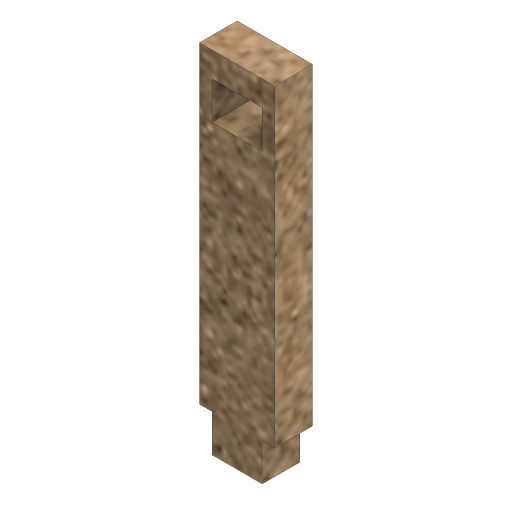
# Autodesk Inventor part: final_side
Saved by Autodesk Inventor 2024 (Build 280153000, 153)
## iProperties
Created: 2024-05-27
Material: MDF Medium Density Fiberboard
Document SubType Name: Modeling
Designer: op04o
Density: 0.8 g/cm^3
Appearance: Cardboard - Corrugated
Mass: 0.36 g
Surface Area: 5.46 cm^2
Volume: 0.45 cm^3
Author: 第26組
Title: final_side
Autodesk Inventor part; units mm, degrees
ref_plane "YZ Plane" through (0, 0, 0) normal (1, 0, 0) x (0, 1, 0)
ref_plane "XZ Plane" through (0, 0, 0) normal (0, 1, 0) x (-1, 0, 0)
ref_plane "XY Plane" through (0, 0, 0) normal (0, 0, 1) x (1, 0, 0)
sketch "Sketch1" plane through (0, 0, 0) normal (0, 0, 1) x (1, 0, 0)
  line L0 (-3, -12.5) -> (3, -12.5)
  line L1 (3, -12.5) -> (3, 12.5)
  line L2 (3, 12.5) -> (-3, 12.5)
  line L3 (-3, 12.5) -> (-3, -12.5)
  line L4 (-3, -12.5) -> (3, 12.5) construction
  line L5 (3, -12.5) -> (-3, 12.5) construction
  line L6 (-2, -12.5) -> (2, -12.5)
  line L7 (2, -12.5) -> (2, -15.5)
  line L8 (2, -15.5) -> (-2, -15.5)
  line L9 (-2, -15.5) -> (-2, -12.5)
  line L10 (-2, 7.5) -> (2, 7.5)
  line L11 (2, 7.5) -> (2, 10.5)
  line L12 (2, 10.5) -> (-2, 10.5)
  line L13 (-2, 10.5) -> (-2, 7.5)
  line L14 (-2, 7.5) -> (2, 10.5) construction
  line L15 (2, 7.5) -> (-2, 10.5) construction
  point P0 (0, 0)
  point P1 (0, -15.5)
  point P2 (0, -12.5)
  point P3 (0, 9)
  point P4 (0, 10.5)
  point P5 (0, 12.5)
  dimension "d0" = 25
  dimension "d1" = 6
  dimension "d2" = 3
  dimension "d3" = 4
  dimension "d6" = 4
  dimension "d7" = 3
  dimension "d8" = 2
  constraints: 32 end point, 8 midpoint, 6 parallel, 3 horizontal, 3 perpendicular, 2 vertical alignment, 1 point on line
  measures "d0" distance of L0.end L1.end
  measures "d1" distance of L1.end L2.end
  measures "d2" distance of L6.end L7.end
  measures "d3" distance of L7.end L8.end
  measures "d6" distance of L11.end L12.end
  measures "d7" distance of L12.end L10.start
  measures "d8" distance between parallel lines of L12 L2
extrude "Extrusion1" add sketch "Sketch1" along normal blind 3
body "Solid1"
